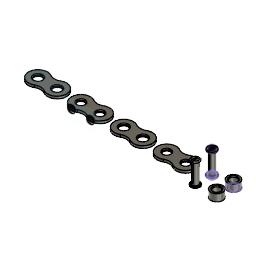
Chain link(barbed pins) (Autodesk Fusion 360 design; units mm, degrees)
part number: 2025-12-20-12-23-50-955
Autodesk Fusion 360 part; units mm, degrees
note: some values were not read from the file. Set by a fixed rule: which sketch regions a step uses.
sketch "Sketch1" plane through (0, 0, 0) normal (0, 0, 1) x (1, 0, 0)
sketch "Sketch2" plane through (0, 0, 0) normal (0, 1, 0) x (1, 0, 0)
  circle A0 centre (0, -0.5) radius 4
  circle A1 centre (8, -0.5) radius 4
  line L0 (1.5, -1.5) -> (2.5, -1.5)
  line L1 (2.5, -1.5) -> (2.5, 0.5)
  line L2 (2.5, 0.5) -> (1.5, 0.5)
  line L3 (1.5, 0.5) -> (1.5, -1.5)
  line L4 (0, -0.5) -> (8, -0.5)
  line L5 (1.5, -2) -> (6.5, -2)
  line L6 (6.5, -2) -> (6.5, 1)
  line L7 (6.5, 1) -> (1.5, 1)
  line L8 (1.5, 1) -> (1.5, -2)
  dimension "d1" = 8
  dimension "d2" = 8
  dimension "d3" = 8
  constraint horizontal L0
  constraint vertical L1
  constraint horizontal L2
  constraint vertical L3
  constraint coincident A0.centre L4.start
  constraint coincident A1.centre L4.end
  constraint horizontal L5
  constraint vertical L6
  constraint horizontal L7
  constraint vertical L8
  measures "d1" distance of A0.centre A1.centre
  measures "d2" diameter of A0
  measures "d3" diameter of A1
extrude "Extrude1" add sketch "Sketch2" against normal blind 1 makes body 1
fillet "Fillet1" radius 4 4 edges at (3.7081, -0.5, 2) (4.2919, -0.5, 2) (3.7081, -0.5, -1) (4.2919, -0.5, -1) on bodies 1
sketch "Sketch3" plane through (0, -1, 0) normal (0, -1, 0) x (1, 0, 0)
  arc A0 (6, -2.9641) -> (6, 3.9641) centre (8, 0.5) ccw
  arc A1 (2, 3.9641) -> (6, 3.9641) centre (4, 7.4282) ccw
  arc A2 (2, 3.9641) -> (2, -2.9641) centre (0, 0.5) ccw
  arc A3 (6, -2.9641) -> (2, -2.9641) centre (4, -6.4282) ccw
  circle A4 centre (8, 0.5) radius 1.65
  circle A5 centre (0, 0.5) radius 1.65
  dimension "d8" = 3.3
  dimension "d9" = 3.3
  constraint concentric A0 A4
  constraint concentric A2 A5
  measures "d8" diameter of A5
  measures "d9" diameter of A4
extrude "Extrude2" cut sketch "Sketch3" against normal blind 1 contours A4 | A5 bodies 1
copy_body "CopyPasteBodies1" bodies 1 makes body 2
move_body "Move1" bodies 2 to x (1, 0, 0) y (0, 1, 0) z (0, 0, 1) at (18, 0, 0)
sketch "Sketch4" plane through (0, -1, 0) normal (0, -1, 0) x (1, 0, 0)
  circle A0 centre (18, 0.5) radius 1.65
  circle A1 centre (26, 0.5) radius 1.65
  arc A2 (20, 3.9641) -> (20, -2.9641) centre (18, 0.5) ccw
  arc A3 (24, -2.9641) -> (20, -2.9641) centre (22, -6.4282) ccw
  arc A4 (24, -2.9641) -> (24, 3.9641) centre (26, 0.5) ccw
  arc A5 (20, 3.9641) -> (24, 3.9641) centre (22, 7.4282) ccw
  circle A6 centre (18, 0.5) radius 1.45
  circle A7 centre (26, 0.5) radius 1.45
  dimension "d12" = 2.9
  dimension "d13" = 2.9
  constraint concentric A0 A6
  constraint concentric A1 A7
  measures "d12" diameter of A7
  measures "d13" diameter of A6
extrude "Extrude3" add sketch "Sketch4" against normal blind 1 contours A0 | A1 bodies 2
sketch "Sketch9" plane through (0, -1, 0) normal (0, -1, 0) x (1, 0, 0)
copy_body "CopyPasteBodies2" bodies 1 2 makes body 3 makes body 4
move_body "Move2" bodies 3 4 to x (1, 0, 0) y (0, 1, 0) z (0, 0, 1) at (36, 0, 0)
move_body "Move3" bodies 4 3 2 1 to x (1, 0, 0) y (0, 0, -1) z (0, 1, 0) at (0, 2.5, -4.5)
move_body "Move4" bodies 4 3 2 1 to x (1, 0, 0) y (0, 1, 0) z (0, 0, 1) at (0, 0, 4.5)
sketch "Sketch5" plane through (0, 0, 0) normal (0, 0, 1) x (1, 0, 0)
  circle A0 centre (80, 5) radius 1.5
  circle A1 centre (80, 5) radius 2.5
  dimension "d16" = 3
  dimension "d17" = 5
  constraint concentric A0 A1
  measures "d16" diameter of A0
  measures "d17" diameter of A1
extrude "Extrude4" add sketch "Sketch5" along normal blind 3 separate body makes body 5
sketch "Sketch6" plane through (0, 0, 0) normal (0, 0, 1) x (1, 0, 0)
  circle A0 centre (71, 5) radius 1.25
  dimension "d20" = 2.5
  measures "d20" diameter of A0
extrude "Extrude5" add sketch "Sketch6" along normal blind 9.5 separate body makes body 6
sketch "Sketch7" plane through (0, 0, 0) normal (0, 0, 1) x (1, 0, 0)
  circle A0 centre (71, 5) radius 1.875
  circle A1 centre (71, 5) radius 1.25
  dimension "d23" = 0
  dimension "d24" = 3.75
  measures "d23" distance of A0.centre A1.centre
  measures "d24" diameter of A0
extrude "Extrude6" add sketch "Sketch7" along normal blind 0.5 bodies 6
fillet "Fillet2" radius 0.25 1 edges at (69.2519, 4.322, 0.5) on bodies 6
fillet "Fillet3" radius 0.3 18 edges at (-1.5383, 3.5967, 1) (-1.5383, 2.4033, 0) (6.4617, 2.4033, 0) (6.4617, 3.5967, 1) (16.6481, 2.4757, 0) (16.6481, 3.5243, 1) (24.6481, 2.4757, 0) (24.6481, 3.5243, 1) (34.4617, 2.4033, 0) (34.4617, 3.5967, 1) (42.4617, 2.4033, 0) (42.4617, 3.5967, 1) (52.6481, 2.4757, 0) (52.6481, 3.5243, 1) (60.6481, 2.4757, 0) (60.6481, 3.5243, 1) (78.6015, 5.5424, 0) (78.6015, 5.5424, 3) on bodies 1 2 3 4 5
sketch "Sketch8" plane through (0, 0, 0) normal (0, 1, 0) x (1, 0, 0)
sketch "Sketch10" plane through (0, 0, 0) normal (0, 0, 1) x (1, 0, 0)
sketch "Sketch11" plane through (0, 0, 0) normal (0, 0, 1) x (1, 0, 0)
  circle A0 centre (80, 5) radius 2.5
  dimension "d33" = 5
  measures "d33" diameter of A0
sketch "Sketch12" plane through (0, 0, 0) normal (0, 1, 0) x (1, 0, 0)
sketch "Sketch13" plane through (0, 0, 0) normal (0, 1, 0) x (1, 0, 0)
sketch "Sketch14" plane through (0, 0, 9.5) normal (0, 0, 1) x (-1, 0, 0)
  circle A0 centre (-71, -5) radius 1.25
  circle A1 centre (-71, -5) radius 1.75
  line L0 (-70.7, -6.7241) -> (-71.3, -6.7241)
  line L1 (-71.3, -6.7241) -> (-71.3, -3.2759)
  line L2 (-71.3, -3.2759) -> (-70.7, -3.2759)
  line L3 (-70.7, -3.2759) -> (-70.7, -6.7241)
  dimension "d34" = 3.5
  dimension "d35" = 0.6
  dimension "d36" = 3.4482
  constraint concentric A0 A1
  constraint horizontal L0
  constraint vertical L1
  constraint horizontal L2
  constraint vertical L3
  constraint coincident A1 L1.end
  constraint coincident A1 L0.start
  constraint coincident A1 L0.end
  measures "d34" diameter of A1
  measures "d35" distance of L0.start L0.end
  measures "d36" distance of L0.end L1.end
extrude "Extrude7" cut sketch "Sketch14" against normal blind 8.5 contours A0 L1 L3 | A0 L1 L2 L3 | A0 L0 L1 L3 | A1 L2 | A1 L0 bodies 6
extrude "Extrude8" add sketch "Sketch14" against normal blind 0.495 contours A0 L3 | A0 A1 L3 | A0 L1 | A0 A1 L1 bodies 6
chamfer "Chamfer1" distance 0.46 angle 45 2 edges at (72.75, 5, 9.5) (69.25, 5, 9.5) measured on face at (72.3865, 4.9571, 9.5) measured on face at (69.7462, 5.0429, 9.5) on bodies 6
chamfer "Chamfer3" distance 0.198 angle 10 2 edges at (72.75, 5, 9.005) (69.25, 5, 9.005) measured on face at (72.5802, 5, 9.005) measured on face at (69.4198, 5, 9.005) on bodies 6
fillet "Fillet5" radius 0.3 2 edges at (70.7, 5, 1) (71.3, 5, 1) on bodies 6
copy_body "CopyPasteBodies4" bodies 5 6 makes body 7 makes body 8
move_body "Move6" bodies 7 8 to x (1, 0, 0) y (0, 1, 0) z (0, 0, 1) at (0, -7, 0)
sketch "Sketch15" plane through (0, 0, 1) normal (0, 0, 1) x (-1, 0, 0)
  circle A0 centre (0, -3) radius 1.95
  arc A1 (-2, -6.4641) -> (-2, 0.4641) centre (0, -3) ccw
  arc A2 (-6, 0.4641) -> (-2, 0.4641) centre (-4, 3.9282) ccw
  arc A3 (-6, 0.4641) -> (-6, -6.4641) centre (-8, -3) ccw
  arc A4 (-2, -6.4641) -> (-6, -6.4641) centre (-4, -9.9282) ccw
  circle A5 centre (-8, -3) radius 1.95
  circle A6 through (-69.25, -5, 8.5) (-71.875, -3.4845, 8.5) (-71.875, -6.5155, 8.5)
  circle A7 through (-69.125, -5, -1) (-71.9375, -3.3762, -1) (-71.9375, -6.6238, -1)
  dimension "d49" = 9.5
equation "d23 = 2.652E-06 mm"
named bodies: "Inner plate", "Outer plate", "Inner plate (1)", "Outer plate (1)", "Roller", "Pin", "Roller (1)", "Pin (1)"
